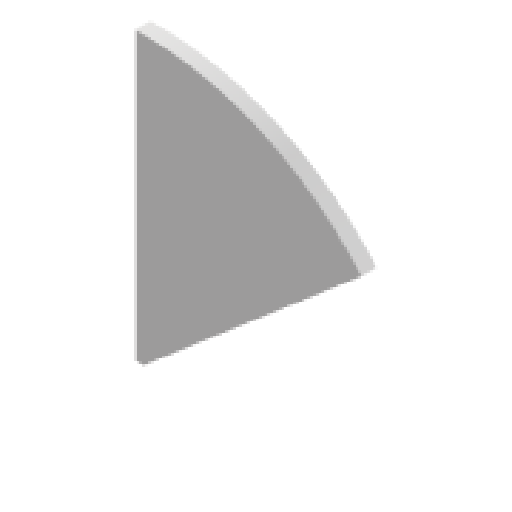
# Autodesk Inventor part: Веер хвоста (сложенный)
Saved by Autodesk Inventor 2023.2 (Build 272271030, 271C)
## iProperties
Created: 2024-03-12
Part Number: Веер хвоста (сложенный)
Material: Типовые
Document SubType Name: Modeling
Designer: I9232
Density: 1 g/cm^3
Appearance: По умолчанию
Author: I9232
Autodesk Inventor part; units mm, degrees
ref_plane "YZ Plane" through (0, 0, 0) normal (1, 0, 0) x (0, 1, 0)
ref_plane "XZ Plane" through (0, 0, 0) normal (0, 1, 0) x (-1, 0, 0)
ref_plane "XY Plane" through (0, 0, 0) normal (0, 0, 1) x (1, 0, 0)
sketch "Эскиз1" plane through (0, 0, 0) normal (0, 0, 1) x (1, 0, 0)
  line L0 (0, -300) -> (18, -300)
  line L1 (18, 300) -> (0, 300)
  line L2 (0, 300) -> (0, -300)
  arc A0 (336.2347, 208.6518) -> (18, 300) centre (18, -300) ccw
  line L3 (18, -300) -> (336.2347, 208.6518)
  point P0 (0, 0)
  dimension "d0" = 600
  dimension "d1" = 18
  dimension "d5" = 18
  constraints: 8 end point, 2 midpoint, 2 point on circle, 1 centre point, 1 coincident, 1 horizontal, 1 parallel, 1 vertical, 1 other
  measures "d0" distance of L0.end L1.start
  measures "d1" distance of L1.start L1.end
  measures "d5" distance of L0.start L0.end
extrude "Выдавливание1" add sketch "Эскиз1" along normal mid plane 32
